Autodesk Inventor part; units mm, degrees
(part 2 of 3)
  circle A1033 centre (-3.85, -0.05) radius 0.15
  circle A1034 centre (-3.85, -0.35) radius 0.15
  circle A1035 centre (-3.85, -0.65) radius 0.15
  circle A1036 centre (-3.85, -0.95) radius 0.15
  circle A1037 centre (-3.85, -1.25) radius 0.15
  circle A1038 centre (-3.85, -1.55) radius 0.15
  circle A1039 centre (-3.85, -1.85) radius 0.15
  circle A1040 centre (-3.85, -2.15) radius 0.15
  circle A1041 centre (-3.85, -2.45) radius 0.15
  circle A1042 centre (-3.85, -2.75) radius 0.15
  circle A1043 centre (-3.85, -3.05) radius 0.15
  circle A1044 centre (-3.85, -3.35) radius 0.15
  circle A1045 centre (-3.85, -3.65) radius 0.15
  circle A1046 centre (-3.85, -3.95) radius 0.15
  circle A1047 centre (-3.85, -4.25) radius 0.15
  circle A1048 centre (-3.85, -4.55) radius 0.15
  circle A1049 centre (-3.85, -4.85) radius 0.15
  circle A1050 centre (-3.55, 9.85) radius 0.15
  circle A1051 centre (-3.55, 9.55) radius 0.15
  circle A1052 centre (-3.55, 9.25) radius 0.15
  circle A1053 centre (-3.55, 8.95) radius 0.15
  circle A1054 centre (-3.55, 8.65) radius 0.15
  circle A1055 centre (-3.55, 8.35) radius 0.15
  circle A1056 centre (-3.55, 8.05) radius 0.15
  circle A1057 centre (-3.55, 7.75) radius 0.15
  circle A1058 centre (-3.55, 7.45) radius 0.15
  circle A1059 centre (-3.55, 7.15) radius 0.15
  circle A1060 centre (-3.55, 6.85) radius 0.15
  circle A1061 centre (-3.55, 6.55) radius 0.15
  circle A1062 centre (-3.55, 6.25) radius 0.15
  circle A1063 centre (-3.55, 5.95) radius 0.15
  circle A1064 centre (-3.55, 5.65) radius 0.15
  circle A1065 centre (-3.55, 5.35) radius 0.15
  circle A1066 centre (-3.55, 5.05) radius 0.15
  circle A1067 centre (-3.55, 4.75) radius 0.15
  circle A1068 centre (-3.55, 4.45) radius 0.15
  circle A1069 centre (-3.55, 4.15) radius 0.15
  circle A1070 centre (-3.55, 3.85) radius 0.15
  circle A1071 centre (-3.55, 3.55) radius 0.15
  circle A1072 centre (-3.55, 3.25) radius 0.15
  circle A1073 centre (-3.55, 2.95) radius 0.15
  circle A1074 centre (-3.55, 2.65) radius 0.15
  circle A1075 centre (-3.55, 2.35) radius 0.15
  circle A1076 centre (-3.55, 2.05) radius 0.15
  circle A1077 centre (-3.55, 1.75) radius 0.15
  circle A1078 centre (-3.55, 1.45) radius 0.15
  circle A1079 centre (-3.55, 1.15) radius 0.15
  circle A1080 centre (-3.55, 0.85) radius 0.15
  circle A1081 centre (-3.55, 0.55) radius 0.15
  circle A1082 centre (-3.55, 0.25) radius 0.15
  circle A1083 centre (-3.55, -0.05) radius 0.15
  circle A1084 centre (-3.55, -0.35) radius 0.15
  circle A1085 centre (-3.55, -0.65) radius 0.15
  circle A1086 centre (-3.55, -0.95) radius 0.15
  circle A1087 centre (-3.55, -1.25) radius 0.15
  circle A1088 centre (-3.55, -1.55) radius 0.15
  circle A1089 centre (-3.55, -1.85) radius 0.15
  circle A1090 centre (-3.55, -2.15) radius 0.15
  circle A1091 centre (-3.55, -2.45) radius 0.15
  circle A1092 centre (-3.55, -2.75) radius 0.15
  circle A1093 centre (-3.55, -3.05) radius 0.15
  circle A1094 centre (-3.55, -3.35) radius 0.15
  circle A1095 centre (-3.55, -3.65) radius 0.15
  circle A1096 centre (-3.55, -3.95) radius 0.15
  circle A1097 centre (-3.55, -4.25) radius 0.15
  circle A1098 centre (-3.55, -4.55) radius 0.15
  circle A1099 centre (-3.55, -4.85) radius 0.15
  circle A1100 centre (-3.25, 9.85) radius 0.15
  circle A1101 centre (-3.25, 9.55) radius 0.15
  circle A1102 centre (-3.25, 9.25) radius 0.15
  circle A1103 centre (-3.25, 8.95) radius 0.15
  circle A1104 centre (-3.25, 8.65) radius 0.15
  circle A1105 centre (-3.25, 8.35) radius 0.15
  circle A1106 centre (-3.25, 8.05) radius 0.15
  circle A1107 centre (-3.25, 7.75) radius 0.15
  circle A1108 centre (-3.25, 7.45) radius 0.15
  circle A1109 centre (-3.25, 7.15) radius 0.15
  circle A1110 centre (-3.25, 6.85) radius 0.15
  circle A1111 centre (-3.25, 6.55) radius 0.15
  circle A1112 centre (-3.25, 6.25) radius 0.15
  circle A1113 centre (-3.25, 5.95) radius 0.15
  circle A1114 centre (-3.25, 5.65) radius 0.15
  circle A1115 centre (-3.25, 5.35) radius 0.15
  circle A1116 centre (-3.25, 5.05) radius 0.15
  circle A1117 centre (-3.25, 4.75) radius 0.15
  circle A1118 centre (-3.25, 4.45) radius 0.15
  circle A1119 centre (-3.25, 4.15) radius 0.15
  circle A1120 centre (-3.25, 3.85) radius 0.15
  circle A1121 centre (-3.25, 3.55) radius 0.15
  circle A1122 centre (-3.25, 3.25) radius 0.15
  circle A1123 centre (-3.25, 2.95) radius 0.15
  circle A1124 centre (-3.25, 2.65) radius 0.15
  circle A1125 centre (-3.25, 2.35) radius 0.15
  circle A1126 centre (-3.25, 2.05) radius 0.15
  circle A1127 centre (-3.25, 1.75) radius 0.15
  circle A1128 centre (-3.25, 1.45) radius 0.15
  circle A1129 centre (-3.25, 1.15) radius 0.15
  circle A1130 centre (-3.25, 0.85) radius 0.15
  circle A1131 centre (-3.25, 0.55) radius 0.15
  circle A1132 centre (-3.25, 0.25) radius 0.15
  circle A1133 centre (-3.25, -0.05) radius 0.15
  circle A1134 centre (-3.25, -0.35) radius 0.15
  circle A1135 centre (-3.25, -0.65) radius 0.15
  circle A1136 centre (-3.25, -0.95) radius 0.15
  circle A1137 centre (-3.25, -1.25) radius 0.15
  circle A1138 centre (-3.25, -1.55) radius 0.15
  circle A1139 centre (-3.25, -1.85) radius 0.15
  circle A1140 centre (-3.25, -2.15) radius 0.15
  circle A1141 centre (-3.25, -2.45) radius 0.15
  circle A1142 centre (-3.25, -2.75) radius 0.15
  circle A1143 centre (-3.25, -3.05) radius 0.15
  circle A1144 centre (-3.25, -3.35) radius 0.15
  circle A1145 centre (-3.25, -3.65) radius 0.15
  circle A1146 centre (-3.25, -3.95) radius 0.15
  circle A1147 centre (-3.25, -4.25) radius 0.15
  circle A1148 centre (-3.25, -4.55) radius 0.15
  circle A1149 centre (-3.25, -4.85) radius 0.15
  circle A1150 centre (-2.95, 9.85) radius 0.15
  circle A1151 centre (-2.95, 9.55) radius 0.15
  circle A1152 centre (-2.95, 9.25) radius 0.15
  circle A1153 centre (-2.95, 8.95) radius 0.15
  circle A1154 centre (-2.95, 8.65) radius 0.15
  circle A1155 centre (-2.95, 8.35) radius 0.15
  circle A1156 centre (-2.95, 8.05) radius 0.15
  circle A1157 centre (-2.95, 7.75) radius 0.15
  circle A1158 centre (-2.95, 7.45) radius 0.15
  circle A1159 centre (-2.95, 7.15) radius 0.15
  circle A1160 centre (-2.95, 6.85) radius 0.15
  circle A1161 centre (-2.95, 6.55) radius 0.15
  circle A1162 centre (-2.95, 6.25) radius 0.15
  circle A1163 centre (-2.95, 5.95) radius 0.15
  circle A1164 centre (-2.95, 5.65) radius 0.15
  circle A1165 centre (-2.95, 5.35) radius 0.15
  circle A1166 centre (-2.95, 5.05) radius 0.15
  circle A1167 centre (-2.95, 4.75) radius 0.15
  circle A1168 centre (-2.95, 4.45) radius 0.15
  circle A1169 centre (-2.95, 4.15) radius 0.15
  circle A1170 centre (-2.95, 3.85) radius 0.15
  circle A1171 centre (-2.95, 3.55) radius 0.15
  circle A1172 centre (-2.95, 3.25) radius 0.15
  circle A1173 centre (-2.95, 2.95) radius 0.15
  circle A1174 centre (-2.95, 2.65) radius 0.15
  circle A1175 centre (-2.95, 2.35) radius 0.15
  circle A1176 centre (-2.95, 2.05) radius 0.15
  circle A1177 centre (-2.95, 1.75) radius 0.15
  circle A1178 centre (-2.95, 1.45) radius 0.15
  circle A1179 centre (-2.95, 1.15) radius 0.15
  circle A1180 centre (-2.95, 0.85) radius 0.15
  circle A1181 centre (-2.95, 0.55) radius 0.15
  circle A1182 centre (-2.95, 0.25) radius 0.15
  circle A1183 centre (-2.95, -0.05) radius 0.15
  circle A1184 centre (-2.95, -0.35) radius 0.15
  circle A1185 centre (-2.95, -0.65) radius 0.15
  circle A1186 centre (-2.95, -0.95) radius 0.15
  circle A1187 centre (-2.95, -1.25) radius 0.15
  circle A1188 centre (-2.95, -1.55) radius 0.15
  circle A1189 centre (-2.95, -1.85) radius 0.15
  circle A1190 centre (-2.95, -2.15) radius 0.15
  circle A1191 centre (-2.95, -2.45) radius 0.15
  circle A1192 centre (-2.95, -2.75) radius 0.15
  circle A1193 centre (-2.95, -3.05) radius 0.15
  circle A1194 centre (-2.95, -3.35) radius 0.15
  circle A1195 centre (-2.95, -3.65) radius 0.15
  circle A1196 centre (-2.95, -3.95) radius 0.15
  circle A1197 centre (-2.95, -4.25) radius 0.15
  circle A1198 centre (-2.95, -4.55) radius 0.15
  circle A1199 centre (-2.95, -4.85) radius 0.15
  circle A1200 centre (-2.65, 9.85) radius 0.15
  circle A1201 centre (-2.65, 9.55) radius 0.15
  circle A1202 centre (-2.65, 9.25) radius 0.15
  circle A1203 centre (-2.65, 8.95) radius 0.15
  circle A1204 centre (-2.65, 8.65) radius 0.15
  circle A1205 centre (-2.65, 8.35) radius 0.15
  circle A1206 centre (-2.65, 8.05) radius 0.15
  circle A1207 centre (-2.65, 7.75) radius 0.15
  circle A1208 centre (-2.65, 7.45) radius 0.15
  circle A1209 centre (-2.65, 7.15) radius 0.15
  circle A1210 centre (-2.65, 6.85) radius 0.15
  circle A1211 centre (-2.65, 6.55) radius 0.15
  circle A1212 centre (-2.65, 6.25) radius 0.15
  circle A1213 centre (-2.65, 5.95) radius 0.15
  circle A1214 centre (-2.65, 5.65) radius 0.15
  circle A1215 centre (-2.65, 5.35) radius 0.15
  circle A1216 centre (-2.65, 5.05) radius 0.15
  circle A1217 centre (-2.65, 4.75) radius 0.15
  circle A1218 centre (-2.65, 4.45) radius 0.15
  circle A1219 centre (-2.65, 4.15) radius 0.15
  circle A1220 centre (-2.65, 3.85) radius 0.15
  circle A1221 centre (-2.65, 3.55) radius 0.15
  circle A1222 centre (-2.65, 3.25) radius 0.15
  circle A1223 centre (-2.65, 2.95) radius 0.15
  circle A1224 centre (-2.65, 2.65) radius 0.15
  circle A1225 centre (-2.65, 2.35) radius 0.15
  circle A1226 centre (-2.65, 2.05) radius 0.15
  circle A1227 centre (-2.65, 1.75) radius 0.15
  circle A1228 centre (-2.65, 1.45) radius 0.15
  circle A1229 centre (-2.65, 1.15) radius 0.15
  circle A1230 centre (-2.65, 0.85) radius 0.15
  circle A1231 centre (-2.65, 0.55) radius 0.15
  circle A1232 centre (-2.65, 0.25) radius 0.15
  circle A1233 centre (-2.65, -0.05) radius 0.15
  circle A1234 centre (-2.65, -0.35) radius 0.15
  circle A1235 centre (-2.65, -0.65) radius 0.15
  circle A1236 centre (-2.65, -0.95) radius 0.15
  circle A1237 centre (-2.65, -1.25) radius 0.15
  circle A1238 centre (-2.65, -1.55) radius 0.15
  circle A1239 centre (-2.65, -1.85) radius 0.15
  circle A1240 centre (-2.65, -2.15) radius 0.15
  circle A1241 centre (-2.65, -2.45) radius 0.15
  circle A1242 centre (-2.65, -2.75) radius 0.15
  circle A1243 centre (-2.65, -3.05) radius 0.15
  circle A1244 centre (-2.65, -3.35) radius 0.15
  circle A1245 centre (-2.65, -3.65) radius 0.15
  circle A1246 centre (-2.65, -3.95) radius 0.15
  circle A1247 centre (-2.65, -4.25) radius 0.15
  circle A1248 centre (-2.65, -4.55) radius 0.15
  circle A1249 centre (-2.65, -4.85) radius 0.15
  circle A1250 centre (-2.35, 9.85) radius 0.15
  circle A1251 centre (-2.35, 9.55) radius 0.15
  circle A1252 centre (-2.35, 9.25) radius 0.15
  circle A1253 centre (-2.35, 8.95) radius 0.15
  circle A1254 centre (-2.35, 8.65) radius 0.15
  circle A1255 centre (-2.35, 8.35) radius 0.15
  circle A1256 centre (-2.35, 8.05) radius 0.15
  circle A1257 centre (-2.35, 7.75) radius 0.15
  circle A1258 centre (-2.35, 7.45) radius 0.15
  circle A1259 centre (-2.35, 7.15) radius 0.15
  circle A1260 centre (-2.35, 6.85) radius 0.15
  circle A1261 centre (-2.35, 6.55) radius 0.15
  circle A1262 centre (-2.35, 6.25) radius 0.15
  circle A1263 centre (-2.35, 5.95) radius 0.15
  circle A1264 centre (-2.35, 5.65) radius 0.15
  circle A1265 centre (-2.35, 5.35) radius 0.15
  circle A1266 centre (-2.35, 5.05) radius 0.15
  circle A1267 centre (-2.35, 4.75) radius 0.15
  circle A1268 centre (-2.35, 4.45) radius 0.15
  circle A1269 centre (-2.35, 4.15) radius 0.15
  circle A1270 centre (-2.35, 3.85) radius 0.15
  circle A1271 centre (-2.35, 3.55) radius 0.15
  circle A1272 centre (-2.35, 3.25) radius 0.15
  circle A1273 centre (-2.35, 2.95) radius 0.15
  circle A1274 centre (-2.35, 2.65) radius 0.15
  circle A1275 centre (-2.35, 2.35) radius 0.15
  circle A1276 centre (-2.35, 2.05) radius 0.15
  circle A1277 centre (-2.35, 1.75) radius 0.15
  circle A1278 centre (-2.35, 1.45) radius 0.15
  circle A1279 centre (-2.35, 1.15) radius 0.15
  circle A1280 centre (-2.35, 0.85) radius 0.15
  circle A1281 centre (-2.35, 0.55) radius 0.15
  circle A1282 centre (-2.35, 0.25) radius 0.15
  circle A1283 centre (-2.35, -0.05) radius 0.15
  circle A1284 centre (-2.35, -0.35) radius 0.15
  circle A1285 centre (-2.35, -0.65) radius 0.15
  circle A1286 centre (-2.35, -0.95) radius 0.15
  circle A1287 centre (-2.35, -1.25) radius 0.15
  circle A1288 centre (-2.35, -1.55) radius 0.15
  circle A1289 centre (-2.35, -1.85) radius 0.15
  circle A1290 centre (-2.35, -2.15) radius 0.15
  circle A1291 centre (-2.35, -2.45) radius 0.15
  circle A1292 centre (-2.35, -2.75) radius 0.15
  circle A1293 centre (-2.35, -3.05) radius 0.15
  circle A1294 centre (-2.35, -3.35) radius 0.15
  circle A1295 centre (-2.35, -3.65) radius 0.15
  circle A1296 centre (-2.35, -3.95) radius 0.15
  circle A1297 centre (-2.35, -4.25) radius 0.15
  circle A1298 centre (-2.35, -4.55) radius 0.15
  circle A1299 centre (-2.35, -4.85) radius 0.15
  circle A1300 centre (-2.05, 9.85) radius 0.15
  circle A1301 centre (-2.05, 9.55) radius 0.15
  circle A1302 centre (-2.05, 9.25) radius 0.15
  circle A1303 centre (-2.05, 8.95) radius 0.15
  circle A1304 centre (-2.05, 8.65) radius 0.15
  circle A1305 centre (-2.05, 8.35) radius 0.15
  circle A1306 centre (-2.05, 8.05) radius 0.15
  circle A1307 centre (-2.05, 7.75) radius 0.15
  circle A1308 centre (-2.05, 7.45) radius 0.15
  circle A1309 centre (-2.05, 7.15) radius 0.15
  circle A1310 centre (-2.05, 6.85) radius 0.15
  circle A1311 centre (-2.05, 6.55) radius 0.15
  circle A1312 centre (-2.05, 6.25) radius 0.15
  circle A1313 centre (-2.05, 5.95) radius 0.15
  circle A1314 centre (-2.05, 5.65) radius 0.15
  circle A1315 centre (-2.05, 5.35) radius 0.15
  circle A1316 centre (-2.05, 5.05) radius 0.15
  circle A1317 centre (-2.05, 4.75) radius 0.15
  circle A1318 centre (-2.05, 4.45) radius 0.15
  circle A1319 centre (-2.05, 4.15) radius 0.15
  circle A1320 centre (-2.05, 3.85) radius 0.15
  circle A1321 centre (-2.05, 3.55) radius 0.15
  circle A1322 centre (-2.05, 3.25) radius 0.15
  circle A1323 centre (-2.05, 2.95) radius 0.15
  circle A1324 centre (-2.05, 2.65) radius 0.15
  circle A1325 centre (-2.05, 2.35) radius 0.15
  circle A1326 centre (-2.05, 2.05) radius 0.15
  circle A1327 centre (-2.05, 1.75) radius 0.15
  circle A1328 centre (-2.05, 1.45) radius 0.15
  circle A1329 centre (-2.05, 1.15) radius 0.15
  circle A1330 centre (-2.05, 0.85) radius 0.15
  circle A1331 centre (-2.05, 0.55) radius 0.15
  circle A1332 centre (-2.05, 0.25) radius 0.15
  circle A1333 centre (-2.05, -0.05) radius 0.15
  circle A1334 centre (-2.05, -0.35) radius 0.15
  circle A1335 centre (-2.05, -0.65) radius 0.15
  circle A1336 centre (-2.05, -0.95) radius 0.15
  circle A1337 centre (-2.05, -1.25) radius 0.15
  circle A1338 centre (-2.05, -1.55) radius 0.15
  circle A1339 centre (-2.05, -1.85) radius 0.15
  circle A1340 centre (-2.05, -2.15) radius 0.15
  circle A1341 centre (-2.05, -2.45) radius 0.15
  circle A1342 centre (-2.05, -2.75) radius 0.15
  circle A1343 centre (-2.05, -3.05) radius 0.15
  circle A1344 centre (-2.05, -3.35) radius 0.15
  circle A1345 centre (-2.05, -3.65) radius 0.15
  circle A1346 centre (-2.05, -3.95) radius 0.15
  circle A1347 centre (-2.05, -4.25) radius 0.15
  circle A1348 centre (-2.05, -4.55) radius 0.15
  circle A1349 centre (-2.05, -4.85) radius 0.15
  circle A1350 centre (-1.75, 9.85) radius 0.15
  circle A1351 centre (-1.75, 9.55) radius 0.15
  circle A1352 centre (-1.75, 9.25) radius 0.15
  circle A1353 centre (-1.75, 8.95) radius 0.15
  circle A1354 centre (-1.75, 8.65) radius 0.15
  circle A1355 centre (-1.75, 8.35) radius 0.15
  circle A1356 centre (-1.75, 8.05) radius 0.15
  circle A1357 centre (-1.75, 7.75) radius 0.15
  circle A1358 centre (-1.75, 7.45) radius 0.15
  circle A1359 centre (-1.75, 7.15) radius 0.15
  circle A1360 centre (-1.75, 6.85) radius 0.15
  circle A1361 centre (-1.75, 6.55) radius 0.15
  circle A1362 centre (-1.75, 6.25) radius 0.15
  circle A1363 centre (-1.75, 5.95) radius 0.15
  circle A1364 centre (-1.75, 5.65) radius 0.15
  circle A1365 centre (-1.75, 5.35) radius 0.15
  circle A1366 centre (-1.75, 5.05) radius 0.15
  circle A1367 centre (-1.75, 4.75) radius 0.15
  circle A1368 centre (-1.75, 4.45) radius 0.15
  circle A1369 centre (-1.75, 4.15) radius 0.15
  circle A1370 centre (-1.75, 3.85) radius 0.15
  circle A1371 centre (-1.75, 3.55) radius 0.15
  circle A1372 centre (-1.75, 3.25) radius 0.15
  circle A1373 centre (-1.75, 2.95) radius 0.15
  circle A1374 centre (-1.75, 2.65) radius 0.15
  circle A1375 centre (-1.75, 2.35) radius 0.15
  circle A1376 centre (-1.75, 2.05) radius 0.15
  circle A1377 centre (-1.75, 1.75) radius 0.15
  circle A1378 centre (-1.75, 1.45) radius 0.15
  circle A1379 centre (-1.75, 1.15) radius 0.15
  circle A1380 centre (-1.75, 0.85) radius 0.15
  circle A1381 centre (-1.75, 0.55) radius 0.15
  circle A1382 centre (-1.75, 0.25) radius 0.15
  circle A1383 centre (-1.75, -0.05) radius 0.15
  circle A1384 centre (-1.75, -0.35) radius 0.15
  circle A1385 centre (-1.75, -0.65) radius 0.15
  circle A1386 centre (-1.75, -0.95) radius 0.15
  circle A1387 centre (-1.75, -1.25) radius 0.15
  circle A1388 centre (-1.75, -1.55) radius 0.15
  circle A1389 centre (-1.75, -1.85) radius 0.15
  circle A1390 centre (-1.75, -2.15) radius 0.15
  circle A1391 centre (-1.75, -2.45) radius 0.15
  circle A1392 centre (-1.75, -2.75) radius 0.15
  circle A1393 centre (-1.75, -3.05) radius 0.15
  circle A1394 centre (-1.75, -3.35) radius 0.15
  circle A1395 centre (-1.75, -3.65) radius 0.15
  circle A1396 centre (-1.75, -3.95) radius 0.15
  circle A1397 centre (-1.75, -4.25) radius 0.15
  circle A1398 centre (-1.75, -4.55) radius 0.15
  circle A1399 centre (-1.75, -4.85) radius 0.15
  circle A1400 centre (-1.45, 9.85) radius 0.15
  circle A1401 centre (-1.45, 9.55) radius 0.15
  circle A1402 centre (-1.45, 9.25) radius 0.15
  circle A1403 centre (-1.45, 8.95) radius 0.15
  circle A1404 centre (-1.45, 8.65) radius 0.15
  circle A1405 centre (-1.45, 8.35) radius 0.15
  circle A1406 centre (-1.45, 8.05) radius 0.15
  circle A1407 centre (-1.45, 7.75) radius 0.15
  circle A1408 centre (-1.45, 7.45) radius 0.15
  circle A1409 centre (-1.45, 7.15) radius 0.15
  circle A1410 centre (-1.45, 6.85) radius 0.15
  circle A1411 centre (-1.45, 6.55) radius 0.15
  circle A1412 centre (-1.45, 6.25) radius 0.15
  circle A1413 centre (-1.45, 5.95) radius 0.15
  circle A1414 centre (-1.45, 5.65) radius 0.15
  circle A1415 centre (-1.45, 5.35) radius 0.15
  circle A1416 centre (-1.45, 5.05) radius 0.15
  circle A1417 centre (-1.45, 4.75) radius 0.15
  circle A1418 centre (-1.45, 4.45) radius 0.15
  circle A1419 centre (-1.45, 4.15) radius 0.15
  circle A1420 centre (-1.45, 3.85) radius 0.15
  circle A1421 centre (-1.45, 3.55) radius 0.15
  circle A1422 centre (-1.45, 3.25) radius 0.15
  circle A1423 centre (-1.45, 2.95) radius 0.15
  circle A1424 centre (-1.45, 2.65) radius 0.15
  circle A1425 centre (-1.45, 2.35) radius 0.15
  circle A1426 centre (-1.45, 2.05) radius 0.15
  circle A1427 centre (-1.45, 1.75) radius 0.15
  circle A1428 centre (-1.45, 1.45) radius 0.15
  circle A1429 centre (-1.45, 1.15) radius 0.15
  circle A1430 centre (-1.45, 0.85) radius 0.15
  circle A1431 centre (-1.45, 0.55) radius 0.15
  circle A1432 centre (-1.45, 0.25) radius 0.15
  circle A1433 centre (-1.45, -0.05) radius 0.15
  circle A1434 centre (-1.45, -0.35) radius 0.15
  circle A1435 centre (-1.45, -0.65) radius 0.15
  circle A1436 centre (-1.45, -0.95) radius 0.15
  circle A1437 centre (-1.45, -1.25) radius 0.15
  circle A1438 centre (-1.45, -1.55) radius 0.15
  circle A1439 centre (-1.45, -1.85) radius 0.15
  circle A1440 centre (-1.45, -2.15) radius 0.15
  circle A1441 centre (-1.45, -2.45) radius 0.15
  circle A1442 centre (-1.45, -2.75) radius 0.15
  circle A1443 centre (-1.45, -3.05) radius 0.15
  circle A1444 centre (-1.45, -3.35) radius 0.15
  circle A1445 centre (-1.45, -3.65) radius 0.15
  circle A1446 centre (-1.45, -3.95) radius 0.15
  circle A1447 centre (-1.45, -4.25) radius 0.15
  circle A1448 centre (-1.45, -4.55) radius 0.15
  circle A1449 centre (-1.45, -4.85) radius 0.15
  circle A1450 centre (-1.15, 9.85) radius 0.15
  circle A1451 centre (-1.15, 9.55) radius 0.15
  circle A1452 centre (-1.15, 9.25) radius 0.15
  circle A1453 centre (-1.15, 8.95) radius 0.15
  circle A1454 centre (-1.15, 8.65) radius 0.15
  circle A1455 centre (-1.15, 8.35) radius 0.15
  circle A1456 centre (-1.15, 8.05) radius 0.15
  circle A1457 centre (-1.15, 7.75) radius 0.15
  circle A1458 centre (-1.15, 7.45) radius 0.15
  circle A1459 centre (-1.15, 7.15) radius 0.15
  circle A1460 centre (-1.15, 6.85) radius 0.15
  circle A1461 centre (-1.15, 6.55) radius 0.15
  circle A1462 centre (-1.15, 6.25) radius 0.15
  circle A1463 centre (-1.15, 5.95) radius 0.15
  circle A1464 centre (-1.15, 5.65) radius 0.15
  circle A1465 centre (-1.15, 5.35) radius 0.15
  circle A1466 centre (-1.15, 5.05) radius 0.15
  circle A1467 centre (-1.15, 4.75) radius 0.15
  circle A1468 centre (-1.15, 4.45) radius 0.15
  circle A1469 centre (-1.15, 4.15) radius 0.15
  circle A1470 centre (-1.15, 3.85) radius 0.15
  circle A1471 centre (-1.15, 3.55) radius 0.15
  circle A1472 centre (-1.15, 3.25) radius 0.15
  circle A1473 centre (-1.15, 2.95) radius 0.15
  circle A1474 centre (-1.15, 2.65) radius 0.15
  circle A1475 centre (-1.15, 2.35) radius 0.15
  circle A1476 centre (-1.15, 2.05) radius 0.15
  circle A1477 centre (-1.15, 1.75) radius 0.15
  circle A1478 centre (-1.15, 1.45) radius 0.15
  circle A1479 centre (-1.15, 1.15) radius 0.15
  circle A1480 centre (-1.15, 0.85) radius 0.15
  circle A1481 centre (-1.15, 0.55) radius 0.15
  circle A1482 centre (-1.15, 0.25) radius 0.15
  circle A1483 centre (-1.15, -0.05) radius 0.15
  circle A1484 centre (-1.15, -0.35) radius 0.15
  circle A1485 centre (-1.15, -0.65) radius 0.15
  circle A1486 centre (-1.15, -0.95) radius 0.15
  circle A1487 centre (-1.15, -1.25) radius 0.15
  circle A1488 centre (-1.15, -1.55) radius 0.15
  circle A1489 centre (-1.15, -1.85) radius 0.15
  circle A1490 centre (-1.15, -2.15) radius 0.15
  circle A1491 centre (-1.15, -2.45) radius 0.15
  circle A1492 centre (-1.15, -2.75) radius 0.15
  circle A1493 centre (-1.15, -3.05) radius 0.15
  circle A1494 centre (-1.15, -3.35) radius 0.15
  circle A1495 centre (-1.15, -3.65) radius 0.15
  circle A1496 centre (-1.15, -3.95) radius 0.15
  circle A1497 centre (-1.15, -4.25) radius 0.15
  circle A1498 centre (-1.15, -4.55) radius 0.15
  circle A1499 centre (-1.15, -4.85) radius 0.15
  circle A1500 centre (-0.85, 9.85) radius 0.15
  circle A1501 centre (-0.85, 9.55) radius 0.15
  circle A1502 centre (-0.85, 9.25) radius 0.15
  circle A1503 centre (-0.85, 8.95) radius 0.15
  circle A1504 centre (-0.85, 8.65) radius 0.15
  circle A1505 centre (-0.85, 8.35) radius 0.15
  circle A1506 centre (-0.85, 8.05) radius 0.15
  circle A1507 centre (-0.85, 7.75) radius 0.15
  circle A1508 centre (-0.85, 7.45) radius 0.15
  circle A1509 centre (-0.85, 7.15) radius 0.15
  circle A1510 centre (-0.85, 6.85) radius 0.15
  circle A1511 centre (-0.85, 6.55) radius 0.15
  circle A1512 centre (-0.85, 6.25) radius 0.15
  circle A1513 centre (-0.85, 5.95) radius 0.15
  circle A1514 centre (-0.85, 5.65) radius 0.15
  circle A1515 centre (-0.85, 5.35) radius 0.15
  circle A1516 centre (-0.85, 5.05) radius 0.15
  circle A1517 centre (-0.85, 4.75) radius 0.15
  circle A1518 centre (-0.85, 4.45) radius 0.15
  circle A1519 centre (-0.85, 4.15) radius 0.15
  circle A1520 centre (-0.85, 3.85) radius 0.15
  circle A1521 centre (-0.85, 3.55) radius 0.15
  circle A1522 centre (-0.85, 3.25) radius 0.15
  circle A1523 centre (-0.85, 2.95) radius 0.15
  circle A1524 centre (-0.85, 2.65) radius 0.15
  circle A1525 centre (-0.85, 2.35) radius 0.15
  circle A1526 centre (-0.85, 2.05) radius 0.15
  circle A1527 centre (-0.85, 1.75) radius 0.15
  circle A1528 centre (-0.85, 1.45) radius 0.15
  circle A1529 centre (-0.85, 1.15) radius 0.15
  circle A1530 centre (-0.85, 0.85) radius 0.15
  circle A1531 centre (-0.85, 0.55) radius 0.15
  circle A1532 centre (-0.85, 0.25) radius 0.15
  circle A1533 centre (-0.85, -0.05) radius 0.15
  circle A1534 centre (-0.85, -0.35) radius 0.15
  circle A1535 centre (-0.85, -0.65) radius 0.15
  circle A1536 centre (-0.85, -0.95) radius 0.15
  circle A1537 centre (-0.85, -1.25) radius 0.15
  circle A1538 centre (-0.85, -1.55) radius 0.15
  circle A1539 centre (-0.85, -1.85) radius 0.15
  circle A1540 centre (-0.85, -2.15) radius 0.15
  circle A1541 centre (-0.85, -2.45) radius 0.15
  circle A1542 centre (-0.85, -2.75) radius 0.15
  circle A1543 centre (-0.85, -3.05) radius 0.15
  circle A1544 centre (-0.85, -3.35) radius 0.15
  circle A1545 centre (-0.85, -3.65) radius 0.15
  circle A1546 centre (-0.85, -3.95) radius 0.15
  circle A1547 centre (-0.85, -4.25) radius 0.15
  circle A1548 centre (-0.85, -4.55) radius 0.15
  circle A1549 centre (-0.85, -4.85) radius 0.15
  circle A1550 centre (-0.55, 9.85) radius 0.15
  circle A1551 centre (-0.55, 9.55) radius 0.15
  circle A1552 centre (-0.55, 9.25) radius 0.15
  circle A1553 centre (-0.55, 8.95) radius 0.15
  circle A1554 centre (-0.55, 8.65) radius 0.15
  circle A1555 centre (-0.55, 8.35) radius 0.15
  circle A1556 centre (-0.55, 8.05) radius 0.15
  circle A1557 centre (-0.55, 7.75) radius 0.15
  circle A1558 centre (-0.55, 7.45) radius 0.15
  circle A1559 centre (-0.55, 7.15) radius 0.15
  circle A1560 centre (-0.55, 6.85) radius 0.15
  circle A1561 centre (-0.55, 6.55) radius 0.15
  circle A1562 centre (-0.55, 6.25) radius 0.15
  circle A1563 centre (-0.55, 5.95) radius 0.15
  circle A1564 centre (-0.55, 5.65) radius 0.15
  circle A1565 centre (-0.55, 5.35) radius 0.15
  circle A1566 centre (-0.55, 5.05) radius 0.15
  circle A1567 centre (-0.55, 4.75) radius 0.15
  circle A1568 centre (-0.55, 4.45) radius 0.15
  circle A1569 centre (-0.55, 4.15) radius 0.15
  circle A1570 centre (-0.55, 3.85) radius 0.15
  circle A1571 centre (-0.55, 3.55) radius 0.15
  circle A1572 centre (-0.55, 3.25) radius 0.15
  circle A1573 centre (-0.55, 2.95) radius 0.15
  circle A1574 centre (-0.55, 2.65) radius 0.15
  circle A1575 centre (-0.55, 2.35) radius 0.15
  circle A1576 centre (-0.55, 2.05) radius 0.15
  circle A1577 centre (-0.55, 1.75) radius 0.15
  circle A1578 centre (-0.55, 1.45) radius 0.15
  circle A1579 centre (-0.55, 1.15) radius 0.15
  circle A1580 centre (-0.55, 0.85) radius 0.15
  circle A1581 centre (-0.55, 0.55) radius 0.15
  circle A1582 centre (-0.55, 0.25) radius 0.15
  circle A1583 centre (-0.55, -0.05) radius 0.15
  circle A1584 centre (-0.55, -0.35) radius 0.15
  circle A1585 centre (-0.55, -0.65) radius 0.15
  circle A1586 centre (-0.55, -0.95) radius 0.15
  circle A1587 centre (-0.55, -1.25) radius 0.15
  circle A1588 centre (-0.55, -1.55) radius 0.15
  circle A1589 centre (-0.55, -1.85) radius 0.15
  circle A1590 centre (-0.55, -2.15) radius 0.15
  circle A1591 centre (-0.55, -2.45) radius 0.15
  circle A1592 centre (-0.55, -2.75) radius 0.15
  circle A1593 centre (-0.55, -3.05) radius 0.15
  circle A1594 centre (-0.55, -3.35) radius 0.15
  circle A1595 centre (-0.55, -3.65) radius 0.15
  circle A1596 centre (-0.55, -3.95) radius 0.15
  circle A1597 centre (-0.55, -4.25) radius 0.15
  circle A1598 centre (-0.55, -4.55) radius 0.15
  circle A1599 centre (-0.55, -4.85) radius 0.15
  circle A1600 centre (-0.25, 9.85) radius 0.15
  circle A1601 centre (-0.25, 9.55) radius 0.15
  circle A1602 centre (-0.25, 9.25) radius 0.15
  circle A1603 centre (-0.25, 8.95) radius 0.15
  circle A1604 centre (-0.25, 8.65) radius 0.15
  circle A1605 centre (-0.25, 8.35) radius 0.15
  circle A1606 centre (-0.25, 8.05) radius 0.15
  circle A1607 centre (-0.25, 7.75) radius 0.15
  circle A1608 centre (-0.25, 7.45) radius 0.15
  circle A1609 centre (-0.25, 7.15) radius 0.15
  circle A1610 centre (-0.25, 6.85) radius 0.15
  circle A1611 centre (-0.25, 6.55) radius 0.15
  circle A1612 centre (-0.25, 6.25) radius 0.15
  circle A1613 centre (-0.25, 5.95) radius 0.15
  circle A1614 centre (-0.25, 5.65) radius 0.15
  circle A1615 centre (-0.25, 5.35) radius 0.15
  circle A1616 centre (-0.25, 5.05) radius 0.15
  circle A1617 centre (-0.25, 4.75) radius 0.15
  circle A1618 centre (-0.25, 4.45) radius 0.15
  circle A1619 centre (-0.25, 4.15) radius 0.15
  circle A1620 centre (-0.25, 3.85) radius 0.15
  circle A1621 centre (-0.25, 3.55) radius 0.15
  circle A1622 centre (-0.25, 3.25) radius 0.15
  circle A1623 centre (-0.25, 2.95) radius 0.15
  circle A1624 centre (-0.25, 2.65) radius 0.15
  circle A1625 centre (-0.25, 2.35) radius 0.15
  circle A1626 centre (-0.25, 2.05) radius 0.15
  circle A1627 centre (-0.25, 1.75) radius 0.15
  circle A1628 centre (-0.25, 1.45) radius 0.15
  circle A1629 centre (-0.25, 1.15) radius 0.15
  circle A1630 centre (-0.25, 0.85) radius 0.15
  circle A1631 centre (-0.25, 0.55) radius 0.15
  circle A1632 centre (-0.25, 0.25) radius 0.15
  circle A1633 centre (-0.25, -0.05) radius 0.15
  circle A1634 centre (-0.25, -0.35) radius 0.15
  circle A1635 centre (-0.25, -0.65) radius 0.15
  circle A1636 centre (-0.25, -0.95) radius 0.15
  circle A1637 centre (-0.25, -1.25) radius 0.15
  circle A1638 centre (-0.25, -1.55) radius 0.15
  circle A1639 centre (-0.25, -1.85) radius 0.15
  circle A1640 centre (-0.25, -2.15) radius 0.15
  circle A1641 centre (-0.25, -2.45) radius 0.15
  circle A1642 centre (-0.25, -2.75) radius 0.15
  circle A1643 centre (-0.25, -3.05) radius 0.15
  circle A1644 centre (-0.25, -3.35) radius 0.15
  circle A1645 centre (-0.25, -3.65) radius 0.15
  circle A1646 centre (-0.25, -3.95) radius 0.15
  circle A1647 centre (-0.25, -4.25) radius 0.15
  circle A1648 centre (-0.25, -4.55) radius 0.15
  circle A1649 centre (-0.25, -4.85) radius 0.15
  circle A1650 centre (0.05, 9.85) radius 0.15
  circle A1651 centre (0.05, 9.55) radius 0.15
  circle A1652 centre (0.05, 9.25) radius 0.15
  circle A1653 centre (0.05, 8.95) radius 0.15
  circle A1654 centre (0.05, 8.65) radius 0.15
  circle A1655 centre (0.05, 8.35) radius 0.15
  circle A1656 centre (0.05, 8.05) radius 0.15
  circle A1657 centre (0.05, 7.75) radius 0.15
  circle A1658 centre (0.05, 7.45) radius 0.15
  circle A1659 centre (0.05, 7.15) radius 0.15
  circle A1660 centre (0.05, 6.85) radius 0.15
  circle A1661 centre (0.05, 6.55) radius 0.15
  circle A1662 centre (0.05, 6.25) radius 0.15
  circle A1663 centre (0.05, 5.95) radius 0.15
  circle A1664 centre (0.05, 5.65) radius 0.15
  circle A1665 centre (0.05, 5.35) radius 0.15
  circle A1666 centre (0.05, 5.05) radius 0.15
  circle A1667 centre (0.05, 4.75) radius 0.15
  circle A1668 centre (0.05, 4.45) radius 0.15
  circle A1669 centre (0.05, 4.15) radius 0.15
  circle A1670 centre (0.05, 3.85) radius 0.15
  circle A1671 centre (0.05, 3.55) radius 0.15
  circle A1672 centre (0.05, 3.25) radius 0.15
  circle A1673 centre (0.05, 2.95) radius 0.15
  circle A1674 centre (0.05, 2.65) radius 0.15
  circle A1675 centre (0.05, 2.35) radius 0.15
  circle A1676 centre (0.05, 2.05) radius 0.15
  circle A1677 centre (0.05, 1.75) radius 0.15
  circle A1678 centre (0.05, 1.45) radius 0.15
  circle A1679 centre (0.05, 1.15) radius 0.15
  circle A1680 centre (0.05, 0.85) radius 0.15
  circle A1681 centre (0.05, 0.55) radius 0.15
  circle A1682 centre (0.05, 0.25) radius 0.15
  circle A1683 centre (0.05, -0.05) radius 0.15
  circle A1684 centre (0.05, -0.35) radius 0.15
  circle A1685 centre (0.05, -0.65) radius 0.15
  circle A1686 centre (0.05, -0.95) radius 0.15
  circle A1687 centre (0.05, -1.25) radius 0.15
  circle A1688 centre (0.05, -1.55) radius 0.15
  circle A1689 centre (0.05, -1.85) radius 0.15
  circle A1690 centre (0.05, -2.15) radius 0.15
  circle A1691 centre (0.05, -2.45) radius 0.15
  circle A1692 centre (0.05, -2.75) radius 0.15
  circle A1693 centre (0.05, -3.05) radius 0.15
  circle A1694 centre (0.05, -3.35) radius 0.15
  circle A1695 centre (0.05, -3.65) radius 0.15
  circle A1696 centre (0.05, -3.95) radius 0.15
  circle A1697 centre (0.05, -4.25) radius 0.15
  circle A1698 centre (0.05, -4.55) radius 0.15
  circle A1699 centre (0.05, -4.85) radius 0.15
  circle A1700 centre (0.35, 9.85) radius 0.15
  circle A1701 centre (0.35, 9.55) radius 0.15
  circle A1702 centre (0.35, 9.25) radius 0.15
  circle A1703 centre (0.35, 8.95) radius 0.15
  circle A1704 centre (0.35, 8.65) radius 0.15
  circle A1705 centre (0.35, 8.35) radius 0.15
  circle A1706 centre (0.35, 8.05) radius 0.15
  circle A1707 centre (0.35, 7.75) radius 0.15
  circle A1708 centre (0.35, 7.45) radius 0.15
  circle A1709 centre (0.35, 7.15) radius 0.15
  circle A1710 centre (0.35, 6.85) radius 0.15
  circle A1711 centre (0.35, 6.55) radius 0.15
  circle A1712 centre (0.35, 6.25) radius 0.15
  circle A1713 centre (0.35, 5.95) radius 0.15
  circle A1714 centre (0.35, 5.65) radius 0.15
  circle A1715 centre (0.35, 5.35) radius 0.15
  circle A1716 centre (0.35, 5.05) radius 0.15
  circle A1717 centre (0.35, 4.75) radius 0.15
  circle A1718 centre (0.35, 4.45) radius 0.15
  circle A1719 centre (0.35, 4.15) radius 0.15
  circle A1720 centre (0.35, 3.85) radius 0.15
  circle A1721 centre (0.35, 3.55) radius 0.15
  circle A1722 centre (0.35, 3.25) radius 0.15
  circle A1723 centre (0.35, 2.95) radius 0.15
  circle A1724 centre (0.35, 2.65) radius 0.15
  circle A1725 centre (0.35, 2.35) radius 0.15
  circle A1726 centre (0.35, 2.05) radius 0.15
  circle A1727 centre (0.35, 1.75) radius 0.15
  circle A1728 centre (0.35, 1.45) radius 0.15
  circle A1729 centre (0.35, 1.15) radius 0.15
  circle A1730 centre (0.35, 0.85) radius 0.15
  circle A1731 centre (0.35, 0.55) radius 0.15
  circle A1732 centre (0.35, 0.25) radius 0.15
  circle A1733 centre (0.35, -0.05) radius 0.15
  circle A1734 centre (0.35, -0.35) radius 0.15
  circle A1735 centre (0.35, -0.65) radius 0.15
  circle A1736 centre (0.35, -0.95) radius 0.15
  circle A1737 centre (0.35, -1.25) radius 0.15
  circle A1738 centre (0.35, -1.55) radius 0.15
  circle A1739 centre (0.35, -1.85) radius 0.15
  circle A1740 centre (0.35, -2.15) radius 0.15
  circle A1741 centre (0.35, -2.45) radius 0.15
  circle A1742 centre (0.35, -2.75) radius 0.15
  circle A1743 centre (0.35, -3.05) radius 0.15
  circle A1744 centre (0.35, -3.35) radius 0.15
  circle A1745 centre (0.35, -3.65) radius 0.15
  circle A1746 centre (0.35, -3.95) radius 0.15
  circle A1747 centre (0.35, -4.25) radius 0.15
  circle A1748 centre (0.35, -4.55) radius 0.15
  circle A1749 centre (0.35, -4.85) radius 0.15
  circle A1750 centre (0.65, 9.85) radius 0.15
  circle A1751 centre (0.65, 9.55) radius 0.15
  circle A1752 centre (0.65, 9.25) radius 0.15
  circle A1753 centre (0.65, 8.95) radius 0.15
  circle A1754 centre (0.65, 8.65) radius 0.15
  circle A1755 centre (0.65, 8.35) radius 0.15
  circle A1756 centre (0.65, 8.05) radius 0.15
  circle A1757 centre (0.65, 7.75) radius 0.15
  circle A1758 centre (0.65, 7.45) radius 0.15
  circle A1759 centre (0.65, 7.15) radius 0.15
  circle A1760 centre (0.65, 6.85) radius 0.15
  circle A1761 centre (0.65, 6.55) radius 0.15
  circle A1762 centre (0.65, 6.25) radius 0.15
  circle A1763 centre (0.65, 5.95) radius 0.15
  circle A1764 centre (0.65, 5.65) radius 0.15
  circle A1765 centre (0.65, 5.35) radius 0.15
  circle A1766 centre (0.65, 5.05) radius 0.15
  circle A1767 centre (0.65, 4.75) radius 0.15
  circle A1768 centre (0.65, 4.45) radius 0.15
  circle A1769 centre (0.65, 4.15) radius 0.15
  circle A1770 centre (0.65, 3.85) radius 0.15
  circle A1771 centre (0.65, 3.55) radius 0.15
  circle A1772 centre (0.65, 3.25) radius 0.15
  circle A1773 centre (0.65, 2.95) radius 0.15
  circle A1774 centre (0.65, 2.65) radius 0.15
  circle A1775 centre (0.65, 2.35) radius 0.15
  circle A1776 centre (0.65, 2.05) radius 0.15
  circle A1777 centre (0.65, 1.75) radius 0.15
  circle A1778 centre (0.65, 1.45) radius 0.15
  circle A1779 centre (0.65, 1.15) radius 0.15
  circle A1780 centre (0.65, 0.85) radius 0.15
  circle A1781 centre (0.65, 0.55) radius 0.15
  circle A1782 centre (0.65, 0.25) radius 0.15
  circle A1783 centre (0.65, -0.05) radius 0.15
  circle A1784 centre (0.65, -0.35) radius 0.15
  circle A1785 centre (0.65, -0.65) radius 0.15
  circle A1786 centre (0.65, -0.95) radius 0.15
  circle A1787 centre (0.65, -1.25) radius 0.15
  circle A1788 centre (0.65, -1.55) radius 0.15
  circle A1789 centre (0.65, -1.85) radius 0.15
  circle A1790 centre (0.65, -2.15) radius 0.15
  circle A1791 centre (0.65, -2.45) radius 0.15
  circle A1792 centre (0.65, -2.75) radius 0.15
  circle A1793 centre (0.65, -3.05) radius 0.15
  circle A1794 centre (0.65, -3.35) radius 0.15
  circle A1795 centre (0.65, -3.65) radius 0.15
  circle A1796 centre (0.65, -3.95) radius 0.15
  circle A1797 centre (0.65, -4.25) radius 0.15
  circle A1798 centre (0.65, -4.55) radius 0.15
  circle A1799 centre (0.65, -4.85) radius 0.15
  circle A1800 centre (0.95, 9.85) radius 0.15
  circle A1801 centre (0.95, 9.55) radius 0.15
  circle A1802 centre (0.95, 9.25) radius 0.15
  circle A1803 centre (0.95, 8.95) radius 0.15
  circle A1804 centre (0.95, 8.65) radius 0.15
  circle A1805 centre (0.95, 8.35) radius 0.15
  circle A1806 centre (0.95, 8.05) radius 0.15
  circle A1807 centre (0.95, 7.75) radius 0.15
  circle A1808 centre (0.95, 7.45) radius 0.15
  circle A1809 centre (0.95, 7.15) radius 0.15
  circle A1810 centre (0.95, 6.85) radius 0.15
  circle A1811 centre (0.95, 6.55) radius 0.15
  circle A1812 centre (0.95, 6.25) radius 0.15
  circle A1813 centre (0.95, 5.95) radius 0.15
  circle A1814 centre (0.95, 5.65) radius 0.15
  circle A1815 centre (0.95, 5.35) radius 0.15
  circle A1816 centre (0.95, 5.05) radius 0.15
  circle A1817 centre (0.95, 4.75) radius 0.15
  circle A1818 centre (0.95, 4.45) radius 0.15
  circle A1819 centre (0.95, 4.15) radius 0.15
  circle A1820 centre (0.95, 3.85) radius 0.15
  circle A1821 centre (0.95, 3.55) radius 0.15
  circle A1822 centre (0.95, 3.25) radius 0.15
  circle A1823 centre (0.95, 2.95) radius 0.15
  circle A1824 centre (0.95, 2.65) radius 0.15
  circle A1825 centre (0.95, 2.35) radius 0.15
  circle A1826 centre (0.95, 2.05) radius 0.15
  circle A1827 centre (0.95, 1.75) radius 0.15
  circle A1828 centre (0.95, 1.45) radius 0.15
  circle A1829 centre (0.95, 1.15) radius 0.15
  circle A1830 centre (0.95, 0.85) radius 0.15
  circle A1831 centre (0.95, 0.55) radius 0.15
  circle A1832 centre (0.95, 0.25) radius 0.15
  circle A1833 centre (0.95, -0.05) radius 0.15
  circle A1834 centre (0.95, -0.35) radius 0.15
  circle A1835 centre (0.95, -0.65) radius 0.15
  circle A1836 centre (0.95, -0.95) radius 0.15
  circle A1837 centre (0.95, -1.25) radius 0.15
  circle A1838 centre (0.95, -1.55) radius 0.15
  circle A1839 centre (0.95, -1.85) radius 0.15
  circle A1840 centre (0.95, -2.15) radius 0.15
  circle A1841 centre (0.95, -2.45) radius 0.15
  circle A1842 centre (0.95, -2.75) radius 0.15
  circle A1843 centre (0.95, -3.05) radius 0.15
  circle A1844 centre (0.95, -3.35) radius 0.15
  circle A1845 centre (0.95, -3.65) radius 0.15
  circle A1846 centre (0.95, -3.95) radius 0.15
  circle A1847 centre (0.95, -4.25) radius 0.15
  circle A1848 centre (0.95, -4.55) radius 0.15
  circle A1849 centre (0.95, -4.85) radius 0.15
  circle A1850 centre (1.25, 9.85) radius 0.15
  circle A1851 centre (1.25, 9.55) radius 0.15
  circle A1852 centre (1.25, 9.25) radius 0.15
  circle A1853 centre (1.25, 8.95) radius 0.15
  circle A1854 centre (1.25, 8.65) radius 0.15
  circle A1855 centre (1.25, 8.35) radius 0.15
  circle A1856 centre (1.25, 8.05) radius 0.15
  circle A1857 centre (1.25, 7.75) radius 0.15
  circle A1858 centre (1.25, 7.45) radius 0.15
  circle A1859 centre (1.25, 7.15) radius 0.15
  circle A1860 centre (1.25, 6.85) radius 0.15
  circle A1861 centre (1.25, 6.55) radius 0.15
  circle A1862 centre (1.25, 6.25) radius 0.15
  circle A1863 centre (1.25, 5.95) radius 0.15
  circle A1864 centre (1.25, 5.65) radius 0.15
  circle A1865 centre (1.25, 5.35) radius 0.15
  circle A1866 centre (1.25, 5.05) radius 0.15
  circle A1867 centre (1.25, 4.75) radius 0.15
  circle A1868 centre (1.25, 4.45) radius 0.15
  circle A1869 centre (1.25, 4.15) radius 0.15
  circle A1870 centre (1.25, 3.85) radius 0.15
  circle A1871 centre (1.25, 3.55) radius 0.15
  circle A1872 centre (1.25, 3.25) radius 0.15
  circle A1873 centre (1.25, 2.95) radius 0.15
  circle A1874 centre (1.25, 2.65) radius 0.15
  circle A1875 centre (1.25, 2.35) radius 0.15
  circle A1876 centre (1.25, 2.05) radius 0.15
  circle A1877 centre (1.25, 1.75) radius 0.15
  circle A1878 centre (1.25, 1.45) radius 0.15
  circle A1879 centre (1.25, 1.15) radius 0.15
  circle A1880 centre (1.25, 0.85) radius 0.15
  circle A1881 centre (1.25, 0.55) radius 0.15
  circle A1882 centre (1.25, 0.25) radius 0.15
  circle A1883 centre (1.25, -0.05) radius 0.15
  circle A1884 centre (1.25, -0.35) radius 0.15
  circle A1885 centre (1.25, -0.65) radius 0.15
  circle A1886 centre (1.25, -0.95) radius 0.15
  circle A1887 centre (1.25, -1.25) radius 0.15
  circle A1888 centre (1.25, -1.55) radius 0.15
  circle A1889 centre (1.25, -1.85) radius 0.15
  circle A1890 centre (1.25, -2.15) radius 0.15
  circle A1891 centre (1.25, -2.45) radius 0.15
  circle A1892 centre (1.25, -2.75) radius 0.15
  circle A1893 centre (1.25, -3.05) radius 0.15
  circle A1894 centre (1.25, -3.35) radius 0.15
  circle A1895 centre (1.25, -3.65) radius 0.15
  circle A1896 centre (1.25, -3.95) radius 0.15
  circle A1897 centre (1.25, -4.25) radius 0.15
  circle A1898 centre (1.25, -4.55) radius 0.15
  circle A1899 centre (1.25, -4.85) radius 0.15
  circle A1900 centre (1.55, 9.85) radius 0.15
  circle A1901 centre (1.55, 9.55) radius 0.15
  circle A1902 centre (1.55, 9.25) radius 0.15
  circle A1903 centre (1.55, 8.95) radius 0.15
  circle A1904 centre (1.55, 8.65) radius 0.15
  circle A1905 centre (1.55, 8.35) radius 0.15
  circle A1906 centre (1.55, 8.05) radius 0.15
  circle A1907 centre (1.55, 7.75) radius 0.15
  circle A1908 centre (1.55, 7.45) radius 0.15
  circle A1909 centre (1.55, 7.15) radius 0.15
  circle A1910 centre (1.55, 6.85) radius 0.15
  circle A1911 centre (1.55, 6.55) radius 0.15
  circle A1912 centre (1.55, 6.25) radius 0.15
  circle A1913 centre (1.55, 5.95) radius 0.15
  circle A1914 centre (1.55, 5.65) radius 0.15
  circle A1915 centre (1.55, 5.35) radius 0.15
  circle A1916 centre (1.55, 5.05) radius 0.15
  circle A1917 centre (1.55, 4.75) radius 0.15
  circle A1918 centre (1.55, 4.45) radius 0.15
  circle A1919 centre (1.55, 4.15) radius 0.15
  circle A1920 centre (1.55, 3.85) radius 0.15
  circle A1921 centre (1.55, 3.55) radius 0.15
  circle A1922 centre (1.55, 3.25) radius 0.15
  circle A1923 centre (1.55, 2.95) radius 0.15
  circle A1924 centre (1.55, 2.65) radius 0.15
  circle A1925 centre (1.55, 2.35) radius 0.15
  circle A1926 centre (1.55, 2.05) radius 0.15
  circle A1927 centre (1.55, 1.75) radius 0.15
  circle A1928 centre (1.55, 1.45) radius 0.15
  circle A1929 centre (1.55, 1.15) radius 0.15
  circle A1930 centre (1.55, 0.85) radius 0.15
  circle A1931 centre (1.55, 0.55) radius 0.15
  circle A1932 centre (1.55, 0.25) radius 0.15
  circle A1933 centre (1.55, -0.05) radius 0.15
  circle A1934 centre (1.55, -0.35) radius 0.15
  circle A1935 centre (1.55, -0.65) radius 0.15
  circle A1936 centre (1.55, -0.95) radius 0.15
  circle A1937 centre (1.55, -1.25) radius 0.15
  circle A1938 centre (1.55, -1.55) radius 0.15
  circle A1939 centre (1.55, -1.85) radius 0.15
  circle A1940 centre (1.55, -2.15) radius 0.15
  circle A1941 centre (1.55, -2.45) radius 0.15
  circle A1942 centre (1.55, -2.75) radius 0.15
  circle A1943 centre (1.55, -3.05) radius 0.15
  circle A1944 centre (1.55, -3.35) radius 0.15
  circle A1945 centre (1.55, -3.65) radius 0.15
  circle A1946 centre (1.55, -3.95) radius 0.15
  circle A1947 centre (1.55, -4.25) radius 0.15
  circle A1948 centre (1.55, -4.55) radius 0.15
  circle A1949 centre (1.55, -4.85) radius 0.15
  circle A1950 centre (1.85, 9.85) radius 0.15
  circle A1951 centre (1.85, 9.55) radius 0.15
  circle A1952 centre (1.85, 9.25) radius 0.15
  circle A1953 centre (1.85, 8.95) radius 0.15
  circle A1954 centre (1.85, 8.65) radius 0.15
  circle A1955 centre (1.85, 8.35) radius 0.15
  circle A1956 centre (1.85, 8.05) radius 0.15
  circle A1957 centre (1.85, 7.75) radius 0.15
  circle A1958 centre (1.85, 7.45) radius 0.15
  circle A1959 centre (1.85, 7.15) radius 0.15
  circle A1960 centre (1.85, 6.85) radius 0.15
  circle A1961 centre (1.85, 6.55) radius 0.15
  circle A1962 centre (1.85, 6.25) radius 0.15
  circle A1963 centre (1.85, 5.95) radius 0.15
  circle A1964 centre (1.85, 5.65) radius 0.15
  circle A1965 centre (1.85, 5.35) radius 0.15
  circle A1966 centre (1.85, 5.05) radius 0.15
  circle A1967 centre (1.85, 4.75) radius 0.15
  circle A1968 centre (1.85, 4.45) radius 0.15
  circle A1969 centre (1.85, 4.15) radius 0.15
  circle A1970 centre (1.85, 3.85) radius 0.15
  circle A1971 centre (1.85, 3.55) radius 0.15
  circle A1972 centre (1.85, 3.25) radius 0.15
  circle A1973 centre (1.85, 2.95) radius 0.15
  circle A1974 centre (1.85, 2.65) radius 0.15
  circle A1975 centre (1.85, 2.35) radius 0.15
  circle A1976 centre (1.85, 2.05) radius 0.15
  circle A1977 centre (1.85, 1.75) radius 0.15
  circle A1978 centre (1.85, 1.45) radius 0.15
  circle A1979 centre (1.85, 1.15) radius 0.15
  circle A1980 centre (1.85, 0.85) radius 0.15
  circle A1981 centre (1.85, 0.55) radius 0.15
  circle A1982 centre (1.85, 0.25) radius 0.15
  circle A1983 centre (1.85, -0.05) radius 0.15
  circle A1984 centre (1.85, -0.35) radius 0.15
  circle A1985 centre (1.85, -0.65) radius 0.15
  circle A1986 centre (1.85, -0.95) radius 0.15
  circle A1987 centre (1.85, -1.25) radius 0.15
  circle A1988 centre (1.85, -1.55) radius 0.15
  circle A1989 centre (1.85, -1.85) radius 0.15
  circle A1990 centre (1.85, -2.15) radius 0.15
  circle A1991 centre (1.85, -2.45) radius 0.15
  circle A1992 centre (1.85, -2.75) radius 0.15
  circle A1993 centre (1.85, -3.05) radius 0.15
  circle A1994 centre (1.85, -3.35) radius 0.15
  circle A1995 centre (1.85, -3.65) radius 0.15
  circle A1996 centre (1.85, -3.95) radius 0.15
  circle A1997 centre (1.85, -4.25) radius 0.15
  circle A1998 centre (1.85, -4.55) radius 0.15
  circle A1999 centre (1.85, -4.85) radius 0.15
  circle A2000 centre (2.15, 9.85) radius 0.15
  circle A2001 centre (2.15, 9.55) radius 0.15
  circle A2002 centre (2.15, 9.25) radius 0.15
  circle A2003 centre (2.15, 8.95) radius 0.15
  circle A2004 centre (2.15, 8.65) radius 0.15
  circle A2005 centre (2.15, 8.35) radius 0.15
  circle A2006 centre (2.15, 8.05) radius 0.15
  circle A2007 centre (2.15, 7.75) radius 0.15
  circle A2008 centre (2.15, 7.45) radius 0.15
  circle A2009 centre (2.15, 7.15) radius 0.15
  circle A2010 centre (2.15, 6.85) radius 0.15
  circle A2011 centre (2.15, 6.55) radius 0.15
  circle A2012 centre (2.15, 6.25) radius 0.15
  circle A2013 centre (2.15, 5.95) radius 0.15
  circle A2014 centre (2.15, 5.65) radius 0.15
  circle A2015 centre (2.15, 5.35) radius 0.15
  circle A2016 centre (2.15, 5.05) radius 0.15
  circle A2017 centre (2.15, 4.75) radius 0.15
  circle A2018 centre (2.15, 4.45) radius 0.15
  circle A2019 centre (2.15, 4.15) radius 0.15
  circle A2020 centre (2.15, 3.85) radius 0.15
  circle A2021 centre (2.15, 3.55) radius 0.15
  circle A2022 centre (2.15, 3.25) radius 0.15
  circle A2023 centre (2.15, 2.95) radius 0.15
  circle A2024 centre (2.15, 2.65) radius 0.15
  circle A2025 centre (2.15, 2.35) radius 0.15
  circle A2026 centre (2.15, 2.05) radius 0.15
  circle A2027 centre (2.15, 1.75) radius 0.15
  circle A2028 centre (2.15, 1.45) radius 0.15
  circle A2029 centre (2.15, 1.15) radius 0.15
  circle A2030 centre (2.15, 0.85) radius 0.15
  circle A2031 centre (2.15, 0.55) radius 0.15
  circle A2032 centre (2.15, 0.25) radius 0.15
  circle A2033 centre (2.15, -0.05) radius 0.15
  circle A2034 centre (2.15, -0.35) radius 0.15
  circle A2035 centre (2.15, -0.65) radius 0.15
  circle A2036 centre (2.15, -0.95) radius 0.15
  circle A2037 centre (2.15, -1.25) radius 0.15
  circle A2038 centre (2.15, -1.55) radius 0.15
  circle A2039 centre (2.15, -1.85) radius 0.15
  circle A2040 centre (2.15, -2.15) radius 0.15
  circle A2041 centre (2.15, -2.45) radius 0.15
  circle A2042 centre (2.15, -2.75) radius 0.15
  circle A2043 centre (2.15, -3.05) radius 0.15
  circle A2044 centre (2.15, -3.35) radius 0.15
  circle A2045 centre (2.15, -3.65) radius 0.15
  circle A2046 centre (2.15, -3.95) radius 0.15
  circle A2047 centre (2.15, -4.25) radius 0.15
  circle A2048 centre (2.15, -4.55) radius 0.15
  circle A2049 centre (2.15, -4.85) radius 0.15
  circle A2050 centre (2.45, 9.85) radius 0.15
  circle A2051 centre (2.45, 9.55) radius 0.15
  circle A2052 centre (2.45, 9.25) radius 0.15
  circle A2053 centre (2.45, 8.95) radius 0.15
  circle A2054 centre (2.45, 8.65) radius 0.15
  circle A2055 centre (2.45, 8.35) radius 0.15
  circle A2056 centre (2.45, 8.05) radius 0.15
  circle A2057 centre (2.45, 7.75) radius 0.15
  circle A2058 centre (2.45, 7.45) radius 0.15
  circle A2059 centre (2.45, 7.15) radius 0.15
  circle A2060 centre (2.45, 6.85) radius 0.15
  circle A2061 centre (2.45, 6.55) radius 0.15
  circle A2062 centre (2.45, 6.25) radius 0.15
  circle A2063 centre (2.45, 5.95) radius 0.15
  circle A2064 centre (2.45, 5.65) radius 0.15
  circle A2065 centre (2.45, 5.35) radius 0.15
  circle A2066 centre (2.45, 5.05) radius 0.15
  circle A2067 centre (2.45, 4.75) radius 0.15
  circle A2068 centre (2.45, 4.45) radius 0.15
  circle A2069 centre (2.45, 4.15) radius 0.15
  circle A2070 centre (2.45, 3.85) radius 0.15
  circle A2071 centre (2.45, 3.55) radius 0.15
  circle A2072 centre (2.45, 3.25) radius 0.15
  circle A2073 centre (2.45, 2.95) radius 0.15